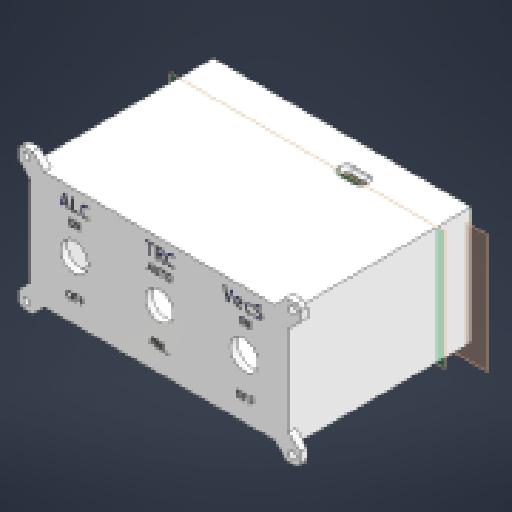
# Autodesk Inventor part: lvl202x01_toggle_body
Saved by Autodesk Inventor 2024 (Build 280153000, 153)
## iProperties
Created: 2026-04-07
Part Number: lvl202x01_toggle_body
Material: ABS Plastic
Document SubType Name: Modeling
Designer: schar
Density: 1.06 g/cm^3
Appearance: Smooth - White
Author: schar
Autodesk Inventor part; units mm, degrees
ref_plane "YZ Plane" through (0, 0, 0) normal (1, 0, 0) x (0, 1, 0)
ref_plane "XZ Plane" through (0, 0, 0) normal (0, 1, 0) x (-1, 0, 0)
ref_plane "XY Plane" through (0, 0, 0) normal (0, 0, 1) x (1, 0, 0)
sketch "Sketch1" plane through (0, 0, 0) normal (0, 0, 1) x (1, 0, 0)
  line L0 (-55, 25) -> (55, 25)
  line L1 (55, 25) -> (55, -25)
  line L2 (55, -25) -> (-55, -25)
  line L3 (-55, -25) -> (-55, 25)
  line L4 (-55, 25) -> (55, -25) construction
  line L5 (55, 25) -> (-55, -25) construction
  line L6 (-55, 25) -> (-49, 25)
  line L7 (-60, 30) -> (60, 30)
  line L8 (60, 30) -> (60, -30)
  line L9 (60, -30) -> (-60, -30)
  line L10 (-60, -30) -> (-60, 30)
  line L11 (-60, 30) -> (60, -30) construction
  line L12 (60, 30) -> (-60, -30) construction
  line L13 (-60, 30) -> (-54, 30)
  line L14 (-54, 30) -> (-49, 25)
  line L15 (-55, 25) -> (-55, 19)
  line L16 (-55, 19) -> (-60, 24)
  circle A0 centre (-56.768, 26.768) radius 1.5 projected
  circle A1 centre (-56.768, 26.768) radius 1.5
  line L17 (55, 25) -> (49, 25)
  line L18 (60, 30) -> (54, 30)
  line L19 (54, 30) -> (49, 25)
  line L20 (55, 25) -> (55, 19)
  line L21 (60, 30) -> (60, 24)
  line L22 (60, 24) -> (55, 19)
  line L23 (55, -25) -> (49, -25)
  line L24 (55, -25) -> (55, -19)
  line L25 (60, -30) -> (60, -24)
  line L26 (60, -30) -> (54, -30)
  line L27 (54, -30) -> (49, -25)
  line L28 (55, -19) -> (60, -24)
  line L29 (-55, -25) -> (-49, -25)
  line L30 (-55, -25) -> (-55, -19)
  line L31 (-60, -30) -> (-60, -24)
  line L32 (-60, -24) -> (-55, -19)
  line L33 (-49, -25) -> (-54, -30)
  circle A2 centre (56.768, 26.768) radius 1.5 projected
  circle A3 centre (56.768, -26.768) radius 1.5 projected
  circle A4 centre (-56.768, -26.768) radius 1.5 projected
  point P0 (0, 0)
  dimension "d0" = 110
  dimension "d1" = 50
  dimension "d2" = 6
  dimension "d3" = 120
  dimension "d4" = 60
  dimension "d5" = 6
  dimension "d6" = 6
  dimension "d7" = 6
  dimension "d8" = 6
  dimension "d9" = 6
  dimension "d10" = 6
  dimension "d11" = 6
  dimension "d12" = 6
  dimension "d13" = 6
  dimension "d14" = 6
  dimension "d15" = 6
  dimension "d16" = 6
  constraints: 68 end point, 16 point on line, 6 parallel, 4 midpoint, 2 horizontal, 2 perpendicular, 1 centre point, 1 coincident, 1 concentric
  measures "d0" distance of L1.end L2.end
  measures "d1" distance of L0.end L1.end
  measures "d2" distance of L0.start L6.end
  measures "d3" distance of L8.end L9.end
  measures "d4" distance of L7.end L8.end
  measures "d5" distance of L7.start L13.end
  measures "d6" distance of L0.end L17.end
  measures "d7" distance of L7.end L18.end
  measures "d8" distance of L0.end L20.end
  measures "d9" distance of L7.end L21.end
  measures "d10" distance of L1.end L23.end
  measures "d11" distance of L1.end L24.end
  measures "d12" distance of L8.end L25.end
  measures "d13" distance of L8.end L26.end
  measures "d14" distance of L2.end L29.end
  measures "d15" distance of L2.end L30.end
  measures "d16" distance of L9.end L31.end
extrude "Extrusion1" add sketch "Sketch1" along normal blind 3 contours L3 L16 L10 L7 L14 L0 | L0 L1 L2 L3 | L19 L7 L8 L22 L1 L0 | L3 L2 L33 L9 L10 L32 | L28 L8 L9 L27 L2 L1
sketch "Sketch2" plane through (0, 0, 0) normal (0, 0, -1) x (-1, 0, 0)
  line L0 (-55, 25) -> (55, 25)
  line L1 (55, 25) -> (55, -25)
  line L2 (55, -25) -> (-55, -25)
  line L3 (-55, -25) -> (-55, 25)
  line L4 (-55, 25) -> (55, -25) construction
  line L5 (55, 25) -> (-55, -25) construction
  line L6 (-55, 25) -> (55, 25)
  line L7 (55, 25) -> (55, -25)
  line L8 (55, -25) -> (-55, -25)
  line L9 (-55, -25) -> (-55, 25)
  line L10 (-55, 25) -> (55, -25) construction
  line L11 (55, 25) -> (-55, -25) construction
  line L12 (-53.2, 23.2) -> (53.2, 23.2)
  line L13 (53.2, 23.2) -> (53.2, -23.2)
  line L14 (53.2, -23.2) -> (-53.2, -23.2)
  line L15 (-53.2, -23.2) -> (-53.2, 23.2)
  line L16 (-53.2, 23.2) -> (53.2, -23.2) construction
  line L17 (53.2, 23.2) -> (-53.2, -23.2) construction
  point P0 (0, 0)
  point P1 (-55, -23)
  point P2 (55, -23)
  point P3 (55, 23)
  point P4 (-55, 23)
  point P5 (-53.2, 25)
  point P6 (-53.2, -25)
  point P7 (53.2, -25)
  point P8 (53.2, 25)
  dimension "d19" = 110
  dimension "d20" = 50
  dimension "d21" = 106.4
  dimension "d22" = 46.4
  constraints: 36 end point, 6 midpoint, 6 parallel, 3 horizontal, 3 perpendicular
  measures "d19" distance of L1.end L2.end
  measures "d20" distance of L0.end L1.end
  measures "d21" distance of L13.end L14.end
  measures "d22" distance of L12.end L13.end
extrude "Extrusion2" add sketch "Sketch2" along normal blind 75
ref_plane "Work Plane1" through (0, 0, -60) normal (0, 0, -1) x (-1, 0, 0)
sketch "Sketch8" plane through (0, 0, 0) normal (0, 0, -1) x (-1, 0, 0)
  line L0 (-53.2, 23.2) -> (-53.2, -23.2) projected
  line L1 (-53.2, 0) -> (-36.2, 0)
  line L2 (53.2, 23.2) -> (53.2, -23.2) projected
  line L3 (53.2, 0) -> (36.2, 0)
  circle A0 centre (-36.2, 0) radius 6
  circle A1 centre (36.2, 0) radius 6
  circle A2 centre (0, 0) radius 6
  dimension "d55" = 17
  dimension "d56" = 17
  dimension "d57" = 12
  dimension "d58" = 12
  dimension "d59" = 12
  constraints: 4 end point, 3 centre point, 3 coincident, 2 horizontal, 2 midpoint
  measures "d55" distance of L1.start L1.end
  measures "d56" distance of L3.start L3.end
  measures "d57" diameter of A0
  measures "d58" diameter of A1
  measures "d59" diameter of A2
extrude "Extrusion7" cut sketch "Sketch8" against normal blind 75
fillet "Fillet1" radius 2 4 edges at (-60, 30, 1.5) (60, 30, 1.5) (60, -30, 1.5) (-60, -30, 1.5)
ref_plane "Work Plane2" through (5.9934, -4.5843, -72.5) normal (0, 0, 1) x (1, 0, 0)
sketch "Sketch9" plane through (5.9934, -4.5843, -72.5) normal (0, 0, 1) x (1, 0, 0)
  circle A0 centre (44.0066, 24.5843) radius 1.1 projected
  circle A1 centre (44.0066, -15.4157) radius 1.1 projected
  circle A2 centre (-138.3891, -45.2455) radius 1.1 projected
  circle A3 centre (-55.9934, 24.5843) radius 1.1 projected
  point P0 (-5.9934, 4.5843)
sketch "Sketch10" plane through (5.9934, -4.5843, -72.5) normal (0, 0, 1) x (1, 0, 0)
  line L0 (-59.1934, 27.7843) -> (-59.1934, -18.6157) projected
  line L1 (-59.1934, -18.6157) -> (-53.1934, -18.6157)
  line L2 (-53.1934, -18.6157) -> (-53.1934, -12.6157)
  line L3 (-53.1934, -12.6157) -> (-59.1934, -12.6157)
  line L4 (-59.1934, -12.6157) -> (-59.1934, -18.6157)
  line L5 (-59.1934, 27.7843) -> (-53.1934, 27.7843)
  line L6 (-53.1934, 27.7843) -> (-53.1934, 21.7843)
  line L7 (-53.1934, 21.7843) -> (-59.1934, 21.7843)
  line L8 (-59.1934, 21.7843) -> (-59.1934, 27.7843)
  line L9 (47.2066, 27.7843) -> (41.2066, 27.7843)
  line L10 (41.2066, 27.7843) -> (41.2066, 21.7843)
  line L11 (41.2066, 21.7843) -> (47.2066, 21.7843)
  line L12 (47.2066, 21.7843) -> (47.2066, 27.7843)
  line L13 (47.2066, -18.6157) -> (41.2066, -18.6157)
  line L14 (41.2066, -18.6157) -> (41.2066, -12.6157)
  line L15 (41.2066, -12.6157) -> (47.2066, -12.6157)
  line L16 (47.2066, -12.6157) -> (47.2066, -18.6157)
  point P0 (-5.9934, 4.5843)
  dimension "d63" = 6
  dimension "d64" = 6
  dimension "d65" = 6
  dimension "d66" = 6
  dimension "d67" = 6
  dimension "d68" = 6
  dimension "d69" = 6
  dimension "d70" = 6
  constraints: 32 end point, 8 parallel, 4 horizontal, 4 perpendicular, 2 point on line
  measures "d63" distance of L3.end L2.end
  measures "d64" distance of L2.end L1.end
  measures "d65" distance of L6.end L7.end
  measures "d66" distance of L5.end L6.end
  measures "d67" distance of L11.end L10.end
  measures "d68" distance of L10.end L9.end
  measures "d69" distance of L14.end L15.end
  measures "d70" distance of L13.end L14.end
extrude "Extrusion8" add sketch "Sketch10" along normal blind 3
fillet "Fillet2" radius 2 4 edges at (47.2, 17.2, -71) (-47.2, 17.2, -71) (-47.2, -17.2, -71) (47.2, -17.2, -71)
extrude "Extrusion9" cut sketch "Sketch9" along normal blind 3
sketch "Sketch11" plane through (0, 0, 3) normal (0, 0, 1) x (1, 0, 0)
  line L0 (-42.5293, 21.409) -> (-20.5849, 21.409) construction
  line L1 (-20.5849, 21.409) -> (-20.5849, 10.8218) construction
  line L2 (-20.5849, 10.8218) -> (-42.5293, 10.8218) construction
  line L3 (-42.5293, 10.8218) -> (-42.5293, 21.409) construction
  line L4 (-6.2817, 21.6334) -> (18.738, 21.6334) construction
  line L5 (18.738, 21.6334) -> (18.738, 8.6423) construction
  line L6 (18.738, 8.6423) -> (-6.2817, 8.6423) construction
  line L7 (-6.2817, 8.6423) -> (-6.2817, 21.6334) construction
  line L8 (27.1178, 21.3326) -> (50.0927, 21.3326) construction
  line L9 (50.0927, 21.3326) -> (50.0927, 6.7177) construction
  line L10 (50.0927, 6.7177) -> (27.1178, 6.7177) construction
  line L11 (27.1178, 6.7177) -> (27.1178, 21.3326) construction
  line L12 (-38.8782, 13.5233) -> (-30.304, 13.5233) construction
  line L13 (-30.304, 13.5233) -> (-30.304, 8.6865) construction
  line L14 (-30.304, 8.6865) -> (-38.8782, 8.6865) construction
  line L15 (-38.8782, 8.6865) -> (-38.8782, 13.5233) construction
  line L16 (-39.5494, -13.451) -> (-22.4595, -13.451) construction
  line L17 (-22.4595, -13.451) -> (-22.4595, -25.6381) construction
  line L18 (-22.4595, -25.6381) -> (-39.5494, -25.6381) construction
  line L19 (-39.5494, -25.6381) -> (-39.5494, -13.451) construction
  line L20 (32.6289, -13.9867) -> (49.7188, -13.9867) construction
  line L21 (49.7188, -13.9867) -> (49.7188, -26.1737) construction
  line L22 (49.7188, -26.1737) -> (32.6289, -26.1737) construction
  line L23 (32.6289, -26.1737) -> (32.6289, -13.9867) construction
  line L24 (33.8386, 13.7371) -> (42.4128, 13.7371) construction
  line L25 (42.4128, 13.7371) -> (42.4128, 8.9004) construction
  line L26 (42.4128, 8.9004) -> (33.8386, 8.9004) construction
  line L27 (33.8386, 8.9004) -> (33.8386, 13.7371) construction
  line L28 (-5.2295, 13.9349) -> (11.2301, 13.9349) construction
  line L29 (11.2301, 13.9349) -> (11.2301, 7.5612) construction
  line L30 (11.2301, 7.5612) -> (-5.2295, 7.5612) construction
  line L31 (-5.2295, 7.5612) -> (-5.2295, 13.9349) construction
  line L32 (-3.8987, -13.0307) -> (11.5102, -13.0307) construction
  line L33 (11.5102, -13.0307) -> (11.5102, -23.2567) construction
  line L34 (11.5102, -23.2567) -> (-3.8987, -23.2567) construction
  line L35 (-3.8987, -23.2567) -> (-3.8987, -13.0307) construction
  line L36 (-38.2551, 16.3463) -> (-38.9988, 16.3463)
  line L37 (-38.9988, 16.3463) -> (-39.3438, 17.435)
  line L38 (-39.3438, 17.435) -> (-41.4361, 17.435)
  line L39 (-41.4361, 17.435) -> (-41.7856, 16.3463)
  line L40 (-41.7856, 16.3463) -> (-42.489, 16.3463)
  line L41 (-42.489, 16.3463) -> (-40.8313, 21.3463)
  line L42 (-40.8313, 21.3463) -> (-39.8949, 21.3463)
  line L43 (-39.8949, 21.3463) -> (-38.2551, 16.3463)
  line L44 (-39.5409, 18.0443) -> (-40.3877, 20.7235)
  line L45 (-40.3877, 20.7235) -> (-41.2435, 18.0443)
  line L46 (-41.2435, 18.0443) -> (-39.5409, 18.0443)
  line L47 (-34.4513, 16.3463) -> (-37.3277, 16.3463)
  line L48 (-37.3277, 16.3463) -> (-37.3277, 21.3463)
  line L49 (-37.3277, 21.3463) -> (-36.6332, 21.3463)
  line L50 (-36.6332, 21.3463) -> (-36.6332, 16.9287)
  line L51 (-36.6332, 16.9287) -> (-34.4513, 16.9287)
  line L52 (-34.4513, 16.9287) -> (-34.4513, 16.3463)
  spline S0 degree 2 poles (-30.101, 16.5345) (-30.7013, 16.2836) (-31.3599, 16.2836) knots 0 0 0 1 1 1
  spline S1 degree 2 poles (-31.3599, 16.2836) (-32.4173, 16.2836) (-33.5553, 17.5515) (-33.5553, 18.7925) knots 0 0 0 1 2 2 2
  spline S2 degree 2 poles (-33.5553, 18.7925) (-33.5553, 19.3929) (-33.2417, 20.3651) (-32.6592, 21.0416) (-31.8348, 21.409) (-31.3196, 21.409) knots 0 0 0 1 2 3 4 4 4
  spline S3 degree 2 poles (-31.3196, 21.409) (-30.9746, 21.409) (-30.3743, 21.2881) (-30.101, 21.1671) knots 0 0 0 1 2 2 2
  line L53 (-30.101, 21.1671) -> (-30.101, 20.4995)
  spline S4 degree 2 poles (-30.101, 20.4995) (-30.3743, 20.6474) (-30.9567, 20.8042) (-31.2972, 20.8042) knots 0 0 0 1 2 2 2
  spline S5 degree 2 poles (-31.2972, 20.8042) (-31.6512, 20.8042) (-32.2202, 20.5399) (-32.6189, 20.0381) (-32.834, 19.3167) (-32.834, 18.8508) knots 0 0 0 1 2 3 4 4 4
  spline S6 degree 2 poles (-32.834, 18.8508) (-32.834, 17.8786) (-32.0454, 16.8929) (-31.2838, 16.8929) knots 0 0 0 1 2 2 2
  spline S7 degree 2 poles (-31.2838, 16.8929) (-30.9612, 16.8929) (-30.3743, 17.0408) (-30.101, 17.1752) knots 0 0 0 1 2 2 2
  line L54 (-30.101, 17.1752) -> (-30.101, 16.5345)
  spline S8 degree 2 poles (-36.3775, 11.9764) (-36.3775, 11.5637) (-36.5716, 10.9679) (-36.8995, 10.5771) (-37.3423, 10.3885) (-37.5855, 10.3885) knots 0 0 0 1 2 3 4 4 4
  spline S9 degree 2 poles (-37.5855, 10.3885) (-37.8807, 10.3885) (-38.318, 10.6017) (-38.6049, 11.0035) (-38.7443, 11.5801) (-38.7443, 11.9409) knots 0 0 0 1 2 3 4 4 4
  spline S10 degree 2 poles (-38.7443, 11.9409) (-38.7443, 12.3481) (-38.553, 12.9439) (-38.225, 13.3347) (-37.785, 13.5233) (-37.5391, 13.5233) knots 0 0 0 1 2 3 4 4 4
  spline S11 degree 2 poles (-37.5391, 13.5233) (-37.2466, 13.5233) (-36.8094, 13.3074) (-36.5197, 12.9083) (-36.3775, 12.3344) (-36.3775, 11.9764) knots 0 0 0 1 2 3 4 4 4
  spline S12 degree 2 poles (-36.793, 11.9463) (-36.793, 12.2142) (-36.8777, 12.6596) (-37.0635, 12.9821) (-37.356, 13.1598) (-37.5637, 13.1598) knots 0 0 0 1 2 3 4 4 4
  spline S13 degree 2 poles (-37.5637, 13.1598) (-37.7632, 13.1598) (-38.0529, 12.9712) (-38.2387, 12.646) (-38.3289, 12.2087) (-38.3289, 11.9627) knots 0 0 0 1 2 3 4 4 4
  spline S14 degree 2 poles (-38.3289, 11.9627) (-38.3289, 11.6922) (-38.2442, 11.2467) (-38.0583, 10.9269) (-37.7686, 10.7493) (-37.5637, 10.7493) knots 0 0 0 1 2 3 4 4 4
  spline S15 degree 2 poles (-37.5637, 10.7493) (-37.3642, 10.7493) (-37.0717, 10.9379) (-36.8831, 11.2631) (-36.793, 11.6976) (-36.793, 11.9463) knots 0 0 0 1 2 3 4 4 4
  line L55 (-33.896, 10.4295) -> (-34.459, 10.4295)
  line L56 (-34.459, 10.4295) -> (-35.309, 12.3317)
  line L57 (-35.309, 12.3317) -> (-35.5549, 12.9439)
  line L58 (-35.5549, 12.9439) -> (-35.5549, 11.4052)
  line L59 (-35.5549, 11.4052) -> (-35.5549, 10.4295)
  line L60 (-35.5549, 10.4295) -> (-35.9703, 10.4295)
  line L61 (-35.9703, 10.4295) -> (-35.9703, 13.4795)
  line L62 (-35.9703, 13.4795) -> (-35.4155, 13.4795)
  line L63 (-35.4155, 13.4795) -> (-34.6038, 11.6758)
  line L64 (-34.6038, 11.6758) -> (-34.3114, 10.9789)
  line L65 (-34.3114, 10.9789) -> (-34.3114, 12.6132)
  line L66 (-34.3114, 12.6132) -> (-34.3114, 13.4795)
  line L67 (-34.3114, 13.4795) -> (-33.896, 13.4795)
  line L68 (-33.896, 13.4795) -> (-33.896, 10.4295)
  spline S16 degree 2 poles (-37.0488, -14.9979) (-37.0488, -15.4105) (-37.2428, -16.0063) (-37.5707, -16.3971) (-38.0135, -16.5857) (-38.2567, -16.5857) knots 0 0 0 1 2 3 4 4 4
  spline S17 degree 2 poles (-38.2567, -16.5857) (-38.5519, -16.5857) (-38.9892, -16.3725) (-39.2761, -15.9708) (-39.4155, -15.3941) (-39.4155, -15.0334) knots 0 0 0 1 2 3 4 4 4
  spline S18 degree 2 poles (-39.4155, -15.0334) (-39.4155, -14.6262) (-39.2242, -14.0304) (-38.8962, -13.6396) (-38.4562, -13.451) (-38.2103, -13.451) knots 0 0 0 1 2 3 4 4 4
  spline S19 degree 2 poles (-38.2103, -13.451) (-37.9178, -13.451) (-37.4806, -13.6669) (-37.1909, -14.0659) (-37.0488, -14.6398) (-37.0488, -14.9979) knots 0 0 0 1 2 3 4 4 4
  spline S20 degree 2 poles (-37.4642, -15.0279) (-37.4642, -14.7601) (-37.5489, -14.3146) (-37.7347, -13.9921) (-38.0272, -13.8145) (-38.2349, -13.8145) knots 0 0 0 1 2 3 4 4 4
  spline S21 degree 2 poles (-38.2349, -13.8145) (-38.4344, -13.8145) (-38.7241, -14.0031) (-38.9099, -14.3283) (-39.0001, -14.7656) (-39.0001, -15.0115) knots 0 0 0 1 2 3 4 4 4
  spline S22 degree 2 poles (-39.0001, -15.0115) (-39.0001, -15.2821) (-38.9154, -15.7276) (-38.7295, -16.0473) (-38.4398, -16.225) (-38.2349, -16.225) knots 0 0 0 1 2 3 4 4 4
  spline S23 degree 2 poles (-38.2349, -16.225) (-38.0354, -16.225) (-37.7429, -16.0364) (-37.5544, -15.7112) (-37.4642, -15.2766) (-37.4642, -15.0279) knots 0 0 0 1 2 3 4 4 4
  line L69 (-34.723, -13.85) -> (-36.0184, -13.85)
  line L70 (-36.0184, -13.85) -> (-36.0184, -14.8393)
  line L71 (-36.0184, -14.8393) -> (-34.7913, -14.8393)
  line L72 (-34.7913, -14.8393) -> (-34.7913, -15.1864)
  line L73 (-34.7913, -15.1864) -> (-36.0184, -15.1864)
  line L74 (-36.0184, -15.1864) -> (-36.0184, -16.5447)
  line L75 (-36.0184, -16.5447) -> (-36.442, -16.5447)
  line L76 (-36.442, -16.5447) -> (-36.442, -13.4947)
  line L77 (-36.442, -13.4947) -> (-34.723, -13.4947)
  line L78 (-34.723, -13.4947) -> (-34.723, -13.85)
  line L79 (-32.0939, -13.85) -> (-33.3893, -13.85)
  line L80 (-33.3893, -13.85) -> (-33.3893, -14.8393)
  line L81 (-33.3893, -14.8393) -> (-32.1622, -14.8393)
  line L82 (-32.1622, -14.8393) -> (-32.1622, -15.1864)
  line L83 (-32.1622, -15.1864) -> (-33.3893, -15.1864)
  line L84 (-33.3893, -15.1864) -> (-33.3893, -16.5447)
  line L85 (-33.3893, -16.5447) -> (-33.8129, -16.5447)
  line L86 (-33.8129, -16.5447) -> (-33.8129, -13.4947)
  line L87 (-33.8129, -13.4947) -> (-32.0939, -13.4947)
  line L88 (-32.0939, -13.4947) -> (-32.0939, -13.85)
  line L89 (-1.3844, -16.0807) -> (-1.7916, -16.0807)
  line L90 (-1.7916, -16.0807) -> (-1.8517, -14.1759)
  line L91 (-1.8517, -14.1759) -> (-1.8763, -13.4489)
  line L92 (-1.8763, -13.4489) -> (-2.0184, -13.8725)
  line L93 (-2.0184, -13.8725) -> (-2.4694, -15.0859)
  line L94 (-2.4694, -15.0859) -> (-2.7563, -15.0859)
  line L95 (-2.7563, -15.0859) -> (-3.1854, -13.919)
  line L96 (-3.1854, -13.919) -> (-3.3248, -13.4489)
  line L97 (-3.3248, -13.4489) -> (-3.3357, -14.2087)
  line L98 (-3.3357, -14.2087) -> (-3.3904, -16.0807)
  line L99 (-3.3904, -16.0807) -> (-3.7812, -16.0807)
  line L100 (-3.7812, -16.0807) -> (-3.6309, -13.0307)
  line L101 (-3.6309, -13.0307) -> (-3.1389, -13.0307)
  line L102 (-3.1389, -13.0307) -> (-2.729, -14.1786)
  line L103 (-2.729, -14.1786) -> (-2.5978, -14.5667)
  line L104 (-2.5978, -14.5667) -> (-2.4694, -14.1786)
  line L105 (-2.4694, -14.1786) -> (-2.0376, -13.0307)
  line L106 (-2.0376, -13.0307) -> (-1.532, -13.0307)
  line L107 (-1.532, -13.0307) -> (-1.3844, -16.0807)
  line L108 (1.0835, -16.0807) -> (0.5205, -16.0807)
  line L109 (0.5205, -16.0807) -> (-0.3294, -14.1786)
  line L110 (-0.3294, -14.1786) -> (-0.5754, -13.5664)
  line L111 (-0.5754, -13.5664) -> (-0.5754, -15.1051)
  line L112 (-0.5754, -15.1051) -> (-0.5754, -16.0807)
  line L113 (-0.5754, -16.0807) -> (-0.9908, -16.0807)
  line L114 (-0.9908, -16.0807) -> (-0.9908, -13.0307)
  line L115 (-0.9908, -13.0307) -> (-0.436, -13.0307)
  line L116 (-0.436, -13.0307) -> (0.3757, -14.8345)
  line L117 (0.3757, -14.8345) -> (0.6681, -15.5314)
  line L118 (0.6681, -15.5314) -> (0.6681, -13.8971)
  line L119 (0.6681, -13.8971) -> (0.6681, -13.0307)
  line L120 (0.6681, -13.0307) -> (1.0835, -13.0307)
  line L121 (1.0835, -13.0307) -> (1.0835, -16.0807)
  line L122 (3.658, -16.0807) -> (1.9034, -16.0807)
  line L123 (1.9034, -16.0807) -> (1.9034, -13.0307)
  line L124 (1.9034, -13.0307) -> (2.327, -13.0307)
  line L125 (2.327, -13.0307) -> (2.327, -15.7255)
  line L126 (2.327, -15.7255) -> (3.658, -15.7255)
  line L127 (3.658, -15.7255) -> (3.658, -16.0807)
  line L128 (-2.6222, 10.8412) -> (-3.0759, 10.8412)
  line L129 (-3.0759, 10.8412) -> (-3.2863, 11.5053)
  line L130 (-3.2863, 11.5053) -> (-4.5626, 11.5053)
  line L131 (-4.5626, 11.5053) -> (-4.7758, 10.8412)
  line L132 (-4.7758, 10.8412) -> (-5.2049, 10.8412)
  line L133 (-5.2049, 10.8412) -> (-4.1937, 13.8912)
  line L134 (-4.1937, 13.8912) -> (-3.6225, 13.8912)
  line L135 (-3.6225, 13.8912) -> (-2.6222, 10.8412)
  line L136 (-3.4066, 11.877) -> (-3.9231, 13.5113)
  line L137 (-3.9231, 13.5113) -> (-4.4451, 11.877)
  line L138 (-4.4451, 11.877) -> (-3.4066, 11.877)
  spline S24 degree 2 poles (-0.2254, 11.9043) (-0.2254, 11.6529) (-0.3675, 11.2429) (-0.6436, 10.956) (-1.0426, 10.8002) (-1.3022, 10.8002) knots 0 0 0 1 2 3 4 4 4
  spline S25 degree 2 poles (-1.3022, 10.8002) (-1.5864, 10.8002) (-1.9827, 10.9505) (-2.2314, 11.2238) (-2.3462, 11.6037) (-2.3462, 11.8415) knots 0 0 0 1 2 3 4 4 4
  line L139 (-2.3462, 11.8415) -> (-2.3462, 13.8912)
  line L140 (-2.3462, 13.8912) -> (-1.9308, 13.8912)
  line L141 (-1.9308, 13.8912) -> (-1.9308, 11.8743)
  spline S26 degree 2 poles (-1.9308, 11.8743) (-1.9308, 11.6939) (-1.8625, 11.4233) (-1.7094, 11.2402) (-1.4634, 11.1473) (-1.2858, 11.1473) knots 0 0 0 1 2 3 4 4 4
  spline S27 degree 2 poles (-1.2858, 11.1473) (-0.9551, 11.1473) (-0.6408, 11.5299) (-0.6408, 11.877) knots 0 0 0 1 2 2 2
  line L142 (-0.6408, 11.877) -> (-0.6408, 13.8912)
  line L143 (-0.6408, 13.8912) -> (-0.2254, 13.8912)
  line L144 (-0.2254, 13.8912) -> (-0.2254, 11.9043)
  line L145 (2.4584, 13.5359) -> (1.5538, 13.5359)
  line L146 (1.5538, 13.5359) -> (1.5538, 10.8412)
  line L147 (1.5538, 10.8412) -> (1.1329, 10.8412)
  line L148 (1.1329, 10.8412) -> (1.1329, 13.5359)
  line L149 (1.1329, 13.5359) -> (0.2283, 13.5359)
  line L150 (0.2283, 13.5359) -> (0.2283, 13.8912)
  line L151 (0.2283, 13.8912) -> (2.4584, 13.8912)
  line L152 (2.4584, 13.8912) -> (2.4584, 13.5359)
  spline S28 degree 2 poles (5.1586, 12.3881) (5.1586, 11.9754) (4.9645, 11.3796) (4.6366, 10.9888) (4.1938, 10.8002) (3.9506, 10.8002) knots 0 0 0 1 2 3 4 4 4
  spline S29 degree 2 poles (3.9506, 10.8002) (3.6554, 10.8002) (3.2181, 11.0134) (2.9312, 11.4151) (2.7918, 11.9918) (2.7918, 12.3525) knots 0 0 0 1 2 3 4 4 4
  spline S30 degree 2 poles (2.7918, 12.3525) (2.7918, 12.7597) (2.9831, 13.3555) (3.3111, 13.7463) (3.7511, 13.9349) (3.997, 13.9349) knots 0 0 0 1 2 3 4 4 4
  spline S31 degree 2 poles (3.997, 13.9349) (4.2895, 13.9349) (4.7267, 13.719) (5.0164, 13.32) (5.1586, 12.7461) (5.1586, 12.3881) knots 0 0 0 1 2 3 4 4 4
  spline S32 degree 2 poles (4.7431, 12.358) (4.7431, 12.6258) (4.6584, 13.0713) (4.4726, 13.3938) (4.1801, 13.5714) (3.9724, 13.5714) knots 0 0 0 1 2 3 4 4 4
  spline S33 degree 2 poles (3.9724, 13.5714) (3.7729, 13.5714) (3.4832, 13.3829) (3.2974, 13.0576) (3.2072, 12.6204) (3.2072, 12.3744) knots 0 0 0 1 2 3 4 4 4
  spline S34 degree 2 poles (3.2072, 12.3744) (3.2072, 12.1038) (3.2919, 11.6584) (3.4778, 11.3386) (3.7675, 11.161) (3.9724, 11.161) knots 0 0 0 1 2 3 4 4 4
  spline S35 degree 2 poles (3.9724, 11.161) (4.172, 11.161) (4.4644, 11.3495) (4.653, 11.6748) (4.7431, 12.1093) (4.7431, 12.358) knots 0 0 0 1 2 3 4 4 4
  line L153 (-2.2988, 20.9882) -> (-3.7817, 20.9882)
  line L154 (-3.7817, 20.9882) -> (-3.7817, 16.5706)
  line L155 (-3.7817, 16.5706) -> (-4.4717, 16.5706)
  line L156 (-4.4717, 16.5706) -> (-4.4717, 20.9882)
  line L157 (-4.4717, 20.9882) -> (-5.9547, 20.9882)
  line L158 (-5.9547, 20.9882) -> (-5.9547, 21.5706)
  line L159 (-5.9547, 21.5706) -> (-2.2988, 21.5706)
  line L160 (-2.2988, 21.5706) -> (-2.2988, 20.9882)
  line L161 (2.0516, 16.5706) -> (1.281, 16.5706)
  line L162 (1.281, 16.5706) -> (0.5328, 18.1701)
  spline S36 degree 2 poles (0.5328, 18.1701) (0.4521, 18.3538) (0.2729, 18.5957) (0.0713, 18.7346) (-0.1706, 18.7973) (-0.3185, 18.7973) knots 0 0 0 1 2 3 4 4 4
  line L163 (-0.3185, 18.7973) -> (-0.6411, 18.7973)
  line L164 (-0.6411, 18.7973) -> (-0.6411, 16.5706)
  line L165 (-0.6411, 16.5706) -> (-1.3221, 16.5706)
  line L166 (-1.3221, 16.5706) -> (-1.3221, 21.5706)
  line L167 (-1.3221, 21.5706) -> (0.0175, 21.5706)
  spline S37 degree 2 poles (0.0175, 21.5706) (0.4521, 21.5706) (1.0794, 21.378) (1.4826, 21.033) (1.6708, 20.5491) (1.6708, 20.2534) knots 0 0 0 1 2 3 4 4 4
  spline S38 degree 2 poles (1.6708, 20.2534) (1.6708, 20.0205) (1.5319, 19.6038) (1.2631, 19.2633) (0.8598, 19.0169) (0.6, 18.9542) knots 0 0 0 1 2 3 4 4 4
  spline S39 degree 2 poles (0.6, 18.9542) (0.8106, 18.8825) (1.1063, 18.5196) (1.2586, 18.2149) knots 0 0 0 1 2 2 2
  line L168 (1.2586, 18.2149) -> (2.0516, 16.5706)
  spline S40 degree 2 poles (0.9584, 20.1952) (0.9584, 20.5984) (0.4566, 20.9972) (-0.0004, 20.9972) knots 0 0 0 1 2 2 2
  line L169 (-0.0004, 20.9972) -> (-0.6411, 20.9972)
  line L170 (-0.6411, 20.9972) -> (-0.6411, 19.3439)
  line L171 (-0.6411, 19.3439) -> (-0.09, 19.3439)
  spline S41 degree 2 poles (-0.09, 19.3439) (0.152, 19.3439) (0.5373, 19.4559) (0.8106, 19.671) (0.9584, 19.9891) (0.9584, 20.1952) knots 0 0 0 1 2 3 4 4 4
  spline S42 degree 2 poles (6.1466, 16.7588) (5.5462, 16.5079) (4.8876, 16.5079) knots 0 0 0 1 1 1
  spline S43 degree 2 poles (4.8876, 16.5079) (3.8303, 16.5079) (2.6923, 17.7758) (2.6923, 19.0169) knots 0 0 0 1 2 2 2
  spline S44 degree 2 poles (2.6923, 19.0169) (2.6923, 19.6172) (3.0059, 20.5895) (3.5883, 21.266) (4.4127, 21.6334) (4.9279, 21.6334) knots 0 0 0 1 2 3 4 4 4
  spline S45 degree 2 poles (4.9279, 21.6334) (5.2729, 21.6334) (5.8733, 21.5124) (6.1466, 21.3914) knots 0 0 0 1 2 2 2
  line L172 (6.1466, 21.3914) -> (6.1466, 20.7239)
  spline S46 degree 2 poles (6.1466, 20.7239) (5.8733, 20.8717) (5.2908, 21.0285) (4.9503, 21.0285) knots 0 0 0 1 2 2 2
  spline S47 degree 2 poles (4.9503, 21.0285) (4.5964, 21.0285) (4.0274, 20.7642) (3.6287, 20.2624) (3.4136, 19.5411) (3.4136, 19.0751) knots 0 0 0 1 2 3 4 4 4
  spline S48 degree 2 poles (3.4136, 19.0751) (3.4136, 18.1029) (4.2021, 17.1172) (4.9638, 17.1172) knots 0 0 0 1 2 2 2
  spline S49 degree 2 poles (4.9638, 17.1172) (5.2864, 17.1172) (5.8733, 17.2651) (6.1466, 17.3995) knots 0 0 0 1 2 2 2
  line L173 (6.1466, 17.3995) -> (6.1466, 16.7588)
  line L174 (31.4144, 21.261) -> (29.7119, 16.261)
  line L175 (29.7119, 16.261) -> (28.7934, 16.261)
  line L176 (28.7934, 16.261) -> (27.1357, 21.261)
  line L177 (27.1357, 21.261) -> (27.9019, 21.261)
  line L178 (27.9019, 21.261) -> (28.9816, 17.8918)
  line L179 (28.9816, 17.8918) -> (29.2907, 16.9016)
  line L180 (29.2907, 16.9016) -> (29.6044, 17.8918)
  line L181 (29.6044, 17.8918) -> (30.6841, 21.261)
  line L182 (30.6841, 21.261) -> (31.4144, 21.261)
  spline S50 degree 2 poles (35.2854, 18.3846) (35.2854, 18.2457) (35.2764, 18.0531) (35.2719, 17.9679) knots 0 0 0 1 2 2 2
  line L183 (35.2719, 17.9679) -> (32.5703, 17.9679)
  spline S51 degree 2 poles (32.5703, 17.9679) (32.5703, 17.381) (33.2289, 16.7493) (33.8517, 16.7493) knots 0 0 0 1 2 2 2
  spline S52 degree 2 poles (33.8517, 16.7493) (34.0175, 16.7493) (34.3535, 16.7762) (34.6716, 16.821) (34.9583, 16.8792) (35.0793, 16.9151) knots 0 0 0 1 2 3 4 4 4
  line L184 (35.0793, 16.9151) -> (35.0793, 16.3685)
  spline S53 degree 2 poles (35.0793, 16.3685) (34.806, 16.2923) (34.1205, 16.1938) (33.7531, 16.1938) knots 0 0 0 1 2 2 2
  spline S54 degree 2 poles (33.7531, 16.1938) (33.2603, 16.1938) (32.5479, 16.4626) (32.0954, 16.9688) (31.8759, 17.7081) (31.8759, 18.174) knots 0 0 0 1 2 3 4 4 4
  spline S55 degree 2 poles (31.8759, 18.174) (31.8759, 18.5817) (32.1089, 19.3031) (32.5569, 19.8497) (33.2065, 20.1722) (33.6187, 20.1722) knots 0 0 0 1 2 3 4 4 4
  spline S56 degree 2 poles (33.6187, 20.1722) (34.0219, 20.1722) (34.6447, 19.9214) (35.0658, 19.4554) (35.2854, 18.7968) (35.2854, 18.3846) knots 0 0 0 1 2 3 4 4 4
  spline S57 degree 2 poles (34.5909, 18.4787) (34.6044, 18.7341) (34.4789, 19.1597) (34.2235, 19.4688) (33.8427, 19.6391) (33.5873, 19.6391) knots 0 0 0 1 2 3 4 4 4
  spline S58 degree 2 poles (33.5873, 19.6391) (33.3723, 19.6391) (33.0094, 19.4688) (32.7495, 19.1642) (32.5882, 18.7341) (32.5703, 18.4787) knots 0 0 0 1 2 3 4 4 4
  line L185 (32.5703, 18.4787) -> (34.5909, 18.4787)
  spline S59 degree 2 poles (39.3356, 16.4043) (39.0757, 16.3058) (38.5291, 16.2072) (38.2379, 16.2072) knots 0 0 0 1 2 2 2
  spline S60 degree 2 poles (38.2379, 16.2072) (37.3284, 16.2072) (36.3427, 17.1929) (36.3427, 18.1427) knots 0 0 0 1 2 2 2
  spline S61 degree 2 poles (36.3427, 18.1427) (36.3427, 18.5997) (36.625, 19.3389) (37.1402, 19.8676) (37.8526, 20.1543) (38.2782, 20.1543) knots 0 0 0 1 2 3 4 4 4
  spline S62 degree 2 poles (38.2782, 20.1543) (38.5784, 20.1543) (39.0981, 20.0692) (39.3356, 19.9751) knots 0 0 0 1 2 2 2
  line L186 (39.3356, 19.9751) -> (39.3356, 19.3389)
  spline S63 degree 2 poles (39.3356, 19.3389) (39.0847, 19.4688) (38.5694, 19.5898) (38.2916, 19.5898) knots 0 0 0 1 2 2 2
  spline S64 degree 2 poles (38.2916, 19.5898) (38.0363, 19.5898) (37.5793, 19.3927) (37.2343, 19.0253) (37.0372, 18.4966) (37.0372, 18.1651) knots 0 0 0 1 2 3 4 4 4
  spline S65 degree 2 poles (37.0372, 18.1651) (37.0372, 17.4706) (37.7137, 16.7762) (38.3185, 16.7762) knots 0 0 0 1 2 2 2
  spline S66 degree 2 poles (38.3185, 16.7762) (38.5873, 16.7762) (39.0981, 16.9016) (39.3356, 17.0226) knots 0 0 0 1 2 2 2
  line L187 (39.3356, 17.0226) -> (39.3356, 16.4043)
  spline S67 degree 2 poles (43.8606, 17.6185) (43.8606, 17.2601) (43.5694, 16.7269) (43.0497, 16.3685) (42.3194, 16.1938) (41.8759, 16.1938) knots 0 0 0 1 2 3 4 4 4
  spline S68 degree 2 poles (41.8759, 16.1938) (41.6787, 16.1938) (41.2845, 16.2251) (40.9216, 16.2699) (40.599, 16.3282) (40.4691, 16.364) knots 0 0 0 1 2 3 4 4 4
  line L188 (40.4691, 16.364) -> (40.4691, 17.0226)
  spline S69 degree 2 poles (40.4691, 17.0226) (40.7558, 16.9151) (41.4726, 16.7941) (41.9252, 16.7941) knots 0 0 0 1 2 2 2
  spline S70 degree 2 poles (41.9252, 16.7941) (42.2567, 16.7941) (42.7182, 16.8972) (43.0139, 17.0988) (43.1483, 17.39) (43.1483, 17.5782) knots 0 0 0 1 2 3 4 4 4
  spline S71 degree 2 poles (43.1483, 17.5782) (43.1483, 17.7798) (42.9243, 18.0665) (42.5569, 18.295) (42.0864, 18.4832) (41.5936, 18.6803) (41.1232, 18.9133) (40.7558, 19.2314) (40.5318, 19.6615) (40.5318, 19.9572) knots 0 0 0 1 2 3 4 5 6 7 8 8 8
  spline S72 degree 2 poles (40.5318, 19.9572) (40.5318, 20.2126) (40.7468, 20.7099) (41.1994, 21.0952) (41.9028, 21.3326) (42.3956, 21.3326) knots 0 0 0 1 2 3 4 4 4
  spline S73 degree 2 poles (42.3956, 21.3326) (42.521, 21.3326) (42.8167, 21.3102) (43.1169, 21.2699) (43.4126, 21.2162) (43.5381, 21.1848) knots 0 0 0 1 2 3 4 4 4
  line L189 (43.5381, 21.1848) -> (43.5381, 20.571)
  spline S74 degree 2 poles (43.5381, 20.571) (43.2424, 20.6561) (42.6554, 20.7412) (42.3777, 20.7412) knots 0 0 0 1 2 2 2
  spline S75 degree 2 poles (42.3777, 20.7412) (41.7952, 20.7412) (41.2442, 20.3515) (41.2442, 20.0244) knots 0 0 0 1 2 2 2
  spline S76 degree 2 poles (41.2442, 20.0244) (41.2442, 19.8228) (41.4682, 19.5316) (41.8356, 19.2986) (42.306, 19.1149) (42.7988, 18.9133) (43.2692, 18.6758) (43.6366, 18.3533) (43.8606, 17.9142) (43.8606, 17.6185) knots 0 0 0 1 2 3 4 5 6 7 8 8 8
  spline S77 degree 2 poles (36.3393, 12.1903) (36.3393, 11.7776) (36.1452, 11.1818) (35.8173, 10.791) (35.3745, 10.6024) (35.1313, 10.6024) knots 0 0 0 1 2 3 4 4 4
  spline S78 degree 2 poles (35.1313, 10.6024) (34.8361, 10.6024) (34.3989, 10.8156) (34.1119, 11.2173) (33.9725, 11.794) (33.9725, 12.1547) knots 0 0 0 1 2 3 4 4 4
  spline S79 degree 2 poles (33.9725, 12.1547) (33.9725, 12.562) (34.1638, 13.1577) (34.4918, 13.5486) (34.9318, 13.7371) (35.1778, 13.7371) knots 0 0 0 1 2 3 4 4 4
  spline S80 degree 2 poles (35.1778, 13.7371) (35.4702, 13.7371) (35.9075, 13.5212) (36.1972, 13.1222) (36.3393, 12.5483) (36.3393, 12.1903) knots 0 0 0 1 2 3 4 4 4
  spline S81 degree 2 poles (35.9239, 12.1602) (35.9239, 12.428) (35.8391, 12.8735) (35.6533, 13.196) (35.3609, 13.3736) (35.1532, 13.3736) knots 0 0 0 1 2 3 4 4 4
  spline S82 degree 2 poles (35.1532, 13.3736) (34.9537, 13.3736) (34.664, 13.1851) (34.4781, 12.8598) (34.3879, 12.4226) (34.3879, 12.1766) knots 0 0 0 1 2 3 4 4 4
  spline S83 degree 2 poles (34.3879, 12.1766) (34.3879, 11.906) (34.4727, 11.4606) (34.6585, 11.1408) (34.9482, 10.9632) (35.1532, 10.9632) knots 0 0 0 1 2 3 4 4 4
  spline S84 degree 2 poles (35.1532, 10.9632) (35.3527, 10.9632) (35.6451, 11.1517) (35.8337, 11.477) (35.9239, 11.9115) (35.9239, 12.1602) knots 0 0 0 1 2 3 4 4 4
  line L190 (38.8208, 10.6434) -> (38.2578, 10.6434)
  line L191 (38.2578, 10.6434) -> (37.4079, 12.5456)
  line L192 (37.4079, 12.5456) -> (37.1619, 13.1577)
  line L193 (37.1619, 13.1577) -> (37.1619, 11.6191)
  line L194 (37.1619, 11.6191) -> (37.1619, 10.6434)
  line L195 (37.1619, 10.6434) -> (36.7465, 10.6434)
  line L196 (36.7465, 10.6434) -> (36.7465, 13.6934)
  line L197 (36.7465, 13.6934) -> (37.3013, 13.6934)
  line L198 (37.3013, 13.6934) -> (38.113, 11.8896)
  line L199 (38.113, 11.8896) -> (38.4054, 11.1927)
  line L200 (38.4054, 11.1927) -> (38.4054, 12.827)
  line L201 (38.4054, 12.827) -> (38.4054, 13.6934)
  line L202 (38.4054, 13.6934) -> (38.8208, 13.6934)
  line L203 (38.8208, 13.6934) -> (38.8208, 10.6434)
  spline S85 degree 2 poles (35.1295, -15.5335) (35.1295, -15.9462) (34.9355, -16.542) (34.6075, -16.9328) (34.1648, -17.1214) (33.9216, -17.1214) knots 0 0 0 1 2 3 4 4 4
  spline S86 degree 2 poles (33.9216, -17.1214) (33.6264, -17.1214) (33.1891, -16.9082) (32.9022, -16.5065) (32.7628, -15.9298) (32.7628, -15.5691) knots 0 0 0 1 2 3 4 4 4
  spline S87 degree 2 poles (32.7628, -15.5691) (32.7628, -15.1618) (32.9541, -14.5661) (33.282, -14.1752) (33.7221, -13.9867) (33.968, -13.9867) knots 0 0 0 1 2 3 4 4 4
  spline S88 degree 2 poles (33.968, -13.9867) (34.2604, -13.9867) (34.6977, -14.2026) (34.9874, -14.6016) (35.1295, -15.1755) (35.1295, -15.5335) knots 0 0 0 1 2 3 4 4 4
  spline S89 degree 2 poles (34.7141, -15.5636) (34.7141, -15.2958) (34.6294, -14.8503) (34.4436, -14.5278) (34.1511, -14.3502) (33.9434, -14.3502) knots 0 0 0 1 2 3 4 4 4
  spline S90 degree 2 poles (33.9434, -14.3502) (33.7439, -14.3502) (33.4542, -14.5387) (33.2684, -14.864) (33.1782, -15.3012) (33.1782, -15.5472) knots 0 0 0 1 2 3 4 4 4
  spline S91 degree 2 poles (33.1782, -15.5472) (33.1782, -15.8178) (33.2629, -16.2632) (33.4488, -16.583) (33.7384, -16.7606) (33.9434, -16.7606) knots 0 0 0 1 2 3 4 4 4
  spline S92 degree 2 poles (33.9434, -16.7606) (34.1429, -16.7606) (34.4354, -16.5721) (34.6239, -16.2468) (34.7141, -15.8123) (34.7141, -15.5636) knots 0 0 0 1 2 3 4 4 4
  line L204 (37.4553, -14.3857) -> (36.1599, -14.3857)
  line L205 (36.1599, -14.3857) -> (36.1599, -15.375)
  line L206 (36.1599, -15.375) -> (37.387, -15.375)
  line L207 (37.387, -15.375) -> (37.387, -15.7221)
  line L208 (37.387, -15.7221) -> (36.1599, -15.7221)
  line L209 (36.1599, -15.7221) -> (36.1599, -17.0804)
  line L210 (36.1599, -17.0804) -> (35.7363, -17.0804)
  line L211 (35.7363, -17.0804) -> (35.7363, -14.0304)
  line L212 (35.7363, -14.0304) -> (37.4553, -14.0304)
  line L213 (37.4553, -14.0304) -> (37.4553, -14.3857)
  line L214 (40.0844, -14.3857) -> (38.789, -14.3857)
  line L215 (38.789, -14.3857) -> (38.789, -15.375)
  line L216 (38.789, -15.375) -> (40.0161, -15.375)
  line L217 (40.0161, -15.375) -> (40.0161, -15.7221)
  line L218 (40.0161, -15.7221) -> (38.789, -15.7221)
  line L219 (38.789, -15.7221) -> (38.789, -17.0804)
  line L220 (38.789, -17.0804) -> (38.3654, -17.0804)
  line L221 (38.3654, -17.0804) -> (38.3654, -14.0304)
  line L222 (38.3654, -14.0304) -> (40.0844, -14.0304)
  line L223 (40.0844, -14.0304) -> (40.0844, -14.3857)
  point P0 (0, 0)
  dimension "d0" = 110
  dimension "d1" = 50
  dimension "d2" = 6
  dimension "d3" = 120
  dimension "d4" = 60
  dimension "d5" = 6
  dimension "d6" = 6
  dimension "d7" = 6
  dimension "d8" = 6
  dimension "d9" = 6
  dimension "d10" = 6
  dimension "d11" = 6
  dimension "d12" = 6
  dimension "d13" = 6
  dimension "d14" = 6
  dimension "d15" = 6
  dimension "d16" = 6
  constraints: 18 other
extrude "Extrusion10" cut sketch "Sketch11" against normal blind 0.2
sketch "Sketch12" plane through (-49, 25, 3) normal (0, 1, 0) x (1, 0, 0)
  line L0 (70.19, 66.225) -> (63.81, 66.225) projected
  line L1 (63.9679, 64.475) -> (70.0321, 64.475) projected
  arc A0 (63.81, 66.225) -> (62.53, 64.945) centre (63.81, 64.945) ccw projected
  line L2 (62.53, 64.945) -> (62.53, 64.345) projected
  arc A1 (62.53, 64.345) -> (63.81, 63.065) centre (63.81, 64.345) ccw projected
  arc A2 (71.47, 64.945) -> (70.19, 66.225) centre (70.19, 64.945) ccw projected
  arc A3 (70.19, 63.065) -> (71.47, 64.345) centre (70.19, 64.345) ccw projected
  line L3 (66.505, 63.065) -> (70.19, 63.065) projected
  line L4 (63.81, 63.065) -> (66.495, 63.065) projected
  line L5 (71.47, 64.345) -> (71.47, 64.945) projected
  circle A4 centre (70.19, 64.345) radius 1.28
  circle A5 centre (70.19, 64.945) radius 1.28
  circle A6 centre (63.81, 64.945) radius 1.28
  circle A7 centre (63.81, 64.345) radius 1.28
  line L6 (70.19, 63.065) -> (63.81, 63.065)
  line L7 (70.19, 66.225) -> (63.81, 66.225)
  line L8 (71.47, 64.945) -> (71.47, 64.345)
  line L9 (62.53, 64.945) -> (62.53, 64.345)
  point P0 (49, 3)
  point P1 (71.4343, 64.645)
  point P2 (71.47, 64.945)
  point P3 (62.5657, 64.645)
  point P4 (71.47, 64.945)
  point P5 (71.47, 64.345)
  constraints: 8 end point, 4 coincident, 3 collinear, 3 tangent, 2 centre point, 2 concentric, 1 horizontal, 1 perpendicular, 1 vertical, 6 other
extrude "Extrusion11" cut sketch "Sketch12" against normal up to surface (1.8 mm away)
fillet "Fillet3" radius 1.7 8 edges at (13.9049, 25, -60.4399) (13.53, 25, -61.645) (13.9049, 25, -62.8501) (18, 25, -63.225) (22.0951, 25, -62.8501) (22.47, 25, -61.645) (22.0951, 25, -60.4399) (18, 25, -60.065) inverted yes
sketch "Sketch13" plane through (5.9934, -4.5843, -72.5) normal (0, 0, -1) x (-1, 0, 0)
  line L0 (59.1934, -12.6157) -> (59.1934, -18.6157) projected
  line L1 (59.1934, -18.6157) -> (55.9934, -18.6157)
  line L2 (55.9934, -18.6157) -> (55.9934, -15.4157)
  line L3 (55.9934, -15.4157) -> (59.1934, -15.4157)
  line L4 (59.1934, -15.4157) -> (59.1934, -18.6157)
  circle A0 centre (55.9934, -15.4157) radius 1.1
  point P0 (5.9934, 4.5843)
  dimension "d81" = 3.2
  dimension "d82" = 3.2
  dimension "d83" = 2.2
  constraints: 8 end point, 2 parallel, 1 centre point, 1 coincident, 1 horizontal, 1 perpendicular
  measures "d81" distance of L2.end L3.end
  measures "d82" distance of L1.end L2.end
  measures "d83" diameter of A0
extrude "Extrusion12" cut sketch "Sketch13" against normal blind 10 contours A0 L2 L3 | L3 L2 A0
body "Solid1"
